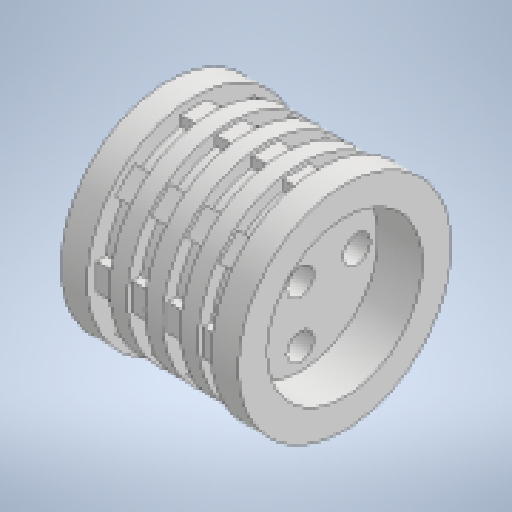
# Autodesk Inventor part: koła tak 1234
Saved by Autodesk Inventor 2023.5 (Build 275446000, 446)
## iProperties
Created: 2025-02-04
Part Number: koła tak 1234
Material: Ogólny
Document SubType Name: Modeling
Designer: idzim
Density: 1 g/cm^3
Appearance: Domyślna
Author: idzim
Autodesk Inventor part; units mm, degrees
ref_plane "YZ Plane" through (0, 0, 0) normal (1, 0, 0) x (0, 1, 0)
ref_plane "XZ Plane" through (0, 0, 0) normal (0, 1, 0) x (-1, 0, 0)
ref_plane "XY Plane" through (0, 0, 0) normal (0, 0, 1) x (1, 0, 0)
sketch "Szkic1" plane through (0, 0, 0) normal (1, 0, 0) x (0, 1, 0)
  circle A0 centre (0, 0) radius 15
  circle A1 centre (0, 0) radius 12
  circle A2 centre (0, 0) radius 10
  circle A3 centre (0, 0) radius 8.75
  dimension "d0" = 30
  dimension "d1" = 24
  dimension "d2" = 20
  dimension "d3" = 17.5
  constraints: 4 centre point, 4 coincident
  measures "d0" diameter of A0
  measures "d1" diameter of A1
  measures "d2" diameter of A2
  measures "d3" diameter of A3
extrude "Wyciągnięcie proste1" add sketch "Szkic1" along normal blind 3 contours A1 | A2 | A3
sketch "Szkic2" plane through (3, 0, 0) normal (1, 0, 0) x (0, 0, -1)
  circle A0 centre (0, 0) radius 8.75
  circle A1 centre (0, 0) radius 10
  circle A2 centre (0, 0) radius 11.25
  line L0 (1.5, 9) -> (-1.5, 9)
  line L1 (-1.5, 9) -> (-1.5, 11)
  line L2 (-1.5, 11) -> (1.5, 11)
  line L3 (1.5, 11) -> (1.5, 9)
  line L4 (1.5, 9) -> (-1.5, 11) construction
  line L5 (-1.5, 9) -> (1.5, 11) construction
  line L6 (-5.3033, 7.4246) -> (-7.4246, 5.3033)
  line L7 (-7.4246, 5.3033) -> (-8.8388, 6.7175)
  line L8 (-8.8388, 6.7175) -> (-6.7175, 8.8388)
  line L9 (-6.7175, 8.8388) -> (-5.3033, 7.4246)
  line L10 (-5.3033, 7.4246) -> (-8.8388, 6.7175) construction
  line L11 (-7.4246, 5.3033) -> (-6.7175, 8.8388) construction
  line L12 (-9, 1.5) -> (-9, -1.5)
  line L13 (-9, -1.5) -> (-11, -1.5)
  line L14 (-11, -1.5) -> (-11, 1.5)
  line L15 (-11, 1.5) -> (-9, 1.5)
  line L16 (-9, 1.5) -> (-11, -1.5) construction
  line L17 (-9, -1.5) -> (-11, 1.5) construction
  line L18 (-7.4246, -5.3033) -> (-5.3033, -7.4246)
  line L19 (-5.3033, -7.4246) -> (-6.7175, -8.8388)
  line L20 (-6.7175, -8.8388) -> (-8.8388, -6.7175)
  line L21 (-8.8388, -6.7175) -> (-7.4246, -5.3033)
  line L22 (-7.4246, -5.3033) -> (-6.7175, -8.8388) construction
  line L23 (-5.3033, -7.4246) -> (-8.8388, -6.7175) construction
  line L24 (-1.5, -9) -> (1.5, -9)
  line L25 (1.5, -9) -> (1.5, -11)
  line L26 (1.5, -11) -> (-1.5, -11)
  line L27 (-1.5, -11) -> (-1.5, -9)
  line L28 (-1.5, -9) -> (1.5, -11) construction
  line L29 (1.5, -9) -> (-1.5, -11) construction
  line L30 (5.3033, -7.4246) -> (7.4246, -5.3033)
  line L31 (7.4246, -5.3033) -> (8.8388, -6.7175)
  line L32 (8.8388, -6.7175) -> (6.7175, -8.8388)
  line L33 (6.7175, -8.8388) -> (5.3033, -7.4246)
  line L34 (5.3033, -7.4246) -> (8.8388, -6.7175) construction
  line L35 (7.4246, -5.3033) -> (6.7175, -8.8388) construction
  line L36 (9, -1.5) -> (9, 1.5)
  line L37 (9, 1.5) -> (11, 1.5)
  line L38 (11, 1.5) -> (11, -1.5)
  line L39 (11, -1.5) -> (9, -1.5)
  line L40 (9, -1.5) -> (11, 1.5) construction
  line L41 (9, 1.5) -> (11, -1.5) construction
  line L42 (7.4246, 5.3033) -> (5.3033, 7.4246)
  line L43 (5.3033, 7.4246) -> (6.7175, 8.8388)
  line L44 (6.7175, 8.8388) -> (8.8388, 6.7175)
  line L45 (8.8388, 6.7175) -> (7.4246, 5.3033)
  line L46 (7.4246, 5.3033) -> (6.7175, 8.8388) construction
  line L47 (5.3033, 7.4246) -> (8.8388, 6.7175) construction
  point P0 (0, 10)
  point P1 (-7.0711, 7.0711)
  point P2 (-10, 0)
  point P3 (-7.0711, -7.0711)
  point P4 (0, -10)
  point P5 (7.0711, -7.0711)
  point P6 (10, 0)
  point P7 (7.0711, 7.0711)
  point P8 (-1.5, 9.8869)
  point P9 (-5.9304, 8.0517)
  point P10 (-8.0517, 5.9304)
  point P11 (-9.8869, 1.5)
  point P12 (-9.8869, -1.5)
  point P13 (-8.0517, -5.9304)
  point P14 (-5.9304, -8.0517)
  point P15 (-1.5, -9.8869)
  point P16 (1.5, -9.8869)
  point P17 (5.9304, -8.0517)
  point P18 (8.0517, -5.9304)
  point P19 (9.8869, -1.5)
  point P20 (9.8869, 1.5)
  point P21 (8.0517, 5.9304)
  point P22 (5.9304, 8.0517)
  point P23 (1.5, 9.8869)
  dimension "d7" = 20
  dimension "d6" = 17.5
  dimension "d8" = 22.5
  dimension "d9" = 3
  dimension "d10" = 2
  dimension "d13" = 360
  constraints: 96 end point, 3 coincident, 2 centre point, 2 midpoint, 2 parallel, 1 horizontal, 1 perpendicular, 92 other
  measures "d6" diameter of A0
  measures "d8" diameter of A2
  measures "d9" distance of L1.end L2.end
  measures "d10" distance of L0.end L1.end
extrude "Wyciągnięcie proste2" add sketch "Szkic2" along normal blind 2 contours A0 | A1 L39 L36 L37 | A1 L37 L38 L39 | L37 L36 L39 A1 L31 L30 L33 L25 L24 L27 L19 L18 L21 L13 L12 L15 L7 L6 L9 L1 L0 L3 L43 L42 L45 | L45 L42 L43 A1 | A1 L43 L44 L45 | L31 L32 L33 A1 | A1 L33 L30 L31 | L3 L0 L1 A1 | A1 L1 L2 L3 | L25 L26 L27 A1 | A1 L27 L24 L25 | L9 L6 L7 A1 | A1 L7 L8 L9 | L19 L20 L21 A1 | A1 L21 L18 L19 | L15 L12 L13 A1 | A1 L13 L14 L15
sketch "Szkic3" plane through (5, 0, 0) normal (1, 0, 0) x (0, 0, -1)
  circle A0 centre (0, 0) radius 11.5
  dimension "d17" = 23
  constraints: 1 centre point, 1 coincident
  measures "d17" diameter of A0
extrude "Wyciągnięcie proste3" add sketch "Szkic3" along normal blind 2
sketch "Szkic4" plane through (7, 0, 0) normal (1, 0, 0) x (0, 0, -1)
  circle A0 centre (0, 0.0528) radius 8.75
  circle A1 centre (0, 0.0528) radius 10
  circle A2 centre (0, 0.0528) radius 11.25
  line L0 (1.5, 9.0528) -> (-1.5, 9.0528)
  line L1 (-1.5, 9.0528) -> (-1.5, 11.0528)
  line L2 (-1.5, 11.0528) -> (1.5, 11.0528)
  line L3 (1.5, 11.0528) -> (1.5, 9.0528)
  line L4 (1.5, 9.0528) -> (-1.5, 11.0528) construction
  line L5 (-1.5, 9.0528) -> (1.5, 11.0528) construction
  line L6 (-5.3033, 7.4774) -> (-7.4246, 5.3561)
  line L7 (-7.4246, 5.3561) -> (-8.8388, 6.7703)
  line L8 (-8.8388, 6.7703) -> (-6.7175, 8.8916)
  line L9 (-6.7175, 8.8916) -> (-5.3033, 7.4774)
  line L10 (-5.3033, 7.4774) -> (-8.8388, 6.7703) construction
  line L11 (-7.4246, 5.3561) -> (-6.7175, 8.8916) construction
  line L12 (-9, 1.5528) -> (-9, -1.4472)
  line L13 (-9, -1.4472) -> (-11, -1.4472)
  line L14 (-11, -1.4472) -> (-11, 1.5528)
  line L15 (-11, 1.5528) -> (-9, 1.5528)
  line L16 (-9, 1.5528) -> (-11, -1.4472) construction
  line L17 (-9, -1.4472) -> (-11, 1.5528) construction
  line L18 (-7.4246, -5.2505) -> (-5.3033, -7.3718)
  line L19 (-5.3033, -7.3718) -> (-6.7175, -8.7861)
  line L20 (-6.7175, -8.7861) -> (-8.8388, -6.6647)
  line L21 (-8.8388, -6.6647) -> (-7.4246, -5.2505)
  line L22 (-7.4246, -5.2505) -> (-6.7175, -8.7861) construction
  line L23 (-5.3033, -7.3718) -> (-8.8388, -6.6647) construction
  line L24 (-1.5, -8.9472) -> (1.5, -8.9472)
  line L25 (1.5, -8.9472) -> (1.5, -10.9472)
  line L26 (1.5, -10.9472) -> (-1.5, -10.9472)
  line L27 (-1.5, -10.9472) -> (-1.5, -8.9472)
  line L28 (-1.5, -8.9472) -> (1.5, -10.9472) construction
  line L29 (1.5, -8.9472) -> (-1.5, -10.9472) construction
  line L30 (5.3033, -7.3718) -> (7.4246, -5.2505)
  line L31 (7.4246, -5.2505) -> (8.8388, -6.6647)
  line L32 (8.8388, -6.6647) -> (6.7175, -8.7861)
  line L33 (6.7175, -8.7861) -> (5.3033, -7.3718)
  line L34 (5.3033, -7.3718) -> (8.8388, -6.6647) construction
  line L35 (7.4246, -5.2505) -> (6.7175, -8.7861) construction
  line L36 (9, -1.4472) -> (9, 1.5528)
  line L37 (9, 1.5528) -> (11, 1.5528)
  line L38 (11, 1.5528) -> (11, -1.4472)
  line L39 (11, -1.4472) -> (9, -1.4472)
  line L40 (9, -1.4472) -> (11, 1.5528) construction
  line L41 (9, 1.5528) -> (11, -1.4472) construction
  line L42 (7.4246, 5.3561) -> (5.3033, 7.4774)
  line L43 (5.3033, 7.4774) -> (6.7175, 8.8916)
  line L44 (6.7175, 8.8916) -> (8.8388, 6.7703)
  line L45 (8.8388, 6.7703) -> (7.4246, 5.3561)
  line L46 (7.4246, 5.3561) -> (6.7175, 8.8916) construction
  line L47 (5.3033, 7.4774) -> (8.8388, 6.7703) construction
  point P0 (0, 0)
  point P1 (0, 10.0528)
  point P2 (-7.0711, 7.1238)
  point P3 (-10, 0.0528)
  point P4 (-7.0711, -7.0183)
  point P5 (0, -9.9472)
  point P6 (7.0711, -7.0183)
  point P7 (10, 0.0528)
  point P8 (7.0711, 7.1238)
  point P9 (-9.8869, -1.4472)
  point P10 (-8.0517, -5.8776)
  point P11 (-5.9304, -7.9989)
  point P12 (-1.5, -9.8341)
  point P13 (1.5, -9.8341)
  point P14 (5.9304, -7.9989)
  point P15 (8.0517, -5.8776)
  point P16 (9.8869, -1.4472)
  point P17 (9.8869, 1.5528)
  point P18 (8.0517, 5.9832)
  point P19 (5.9304, 8.1045)
  point P20 (1.5, 9.9396)
  point P21 (-1.5, 9.9396)
  point P22 (-5.9304, 8.1045)
  point P23 (-8.0517, 5.9832)
  point P24 (-9.8869, 1.5528)
  dimension "d23" = 20
  dimension "d22" = 17.5
  dimension "d24" = 22.5
  dimension "d25" = 3
  dimension "d26" = 2
  dimension "d27" = 360
  constraints: 96 end point, 3 coincident, 2 centre point, 2 midpoint, 2 parallel, 1 horizontal, 1 perpendicular, 92 other
  measures "d22" diameter of A0
  measures "d24" diameter of A2
  measures "d25" distance of L1.end L2.end
  measures "d26" distance of L1.start L1.end
extrude "Wyciągnięcie proste4" add sketch "Szkic4" along normal blind 2 contours A0 | A1 L39 L36 L37 | A1 L37 L38 L39 | L37 L36 L39 A1 L31 L30 L33 L25 L24 L27 L19 L18 L21 L13 L12 L15 L7 L6 L9 L1 L0 L3 L43 L42 L45 | L45 L42 L43 A1 | A1 L43 L44 L45 | L31 L32 L33 A1 | A1 L33 L30 L31 | L3 L0 L1 A1 | A1 L1 L2 L3 | L25 L26 L27 A1 | A1 L27 L24 L25 | L9 L6 L7 A1 | A1 L7 L8 L9 | L19 L20 L21 A1 | A1 L21 L18 L19 | L15 L12 L13 A1 | A1 L13 L14 L15
sketch "Szkic5" plane through (9, 0, 0) normal (1, 0, 0) x (0, 0, -1)
  circle A0 centre (0, 0) radius 11.5
  dimension "d30" = 23
  constraints: 1 centre point, 1 coincident
  measures "d30" diameter of A0
extrude "Wyciągnięcie proste5" add sketch "Szkic5" along normal blind 2
sketch "Szkic6" plane through (11, 0, 0) normal (1, 0, 0) x (0, 0, -1)
  circle A0 centre (0, 0) radius 8.75
  circle A1 centre (0, 0) radius 10
  circle A2 centre (0, 0) radius 11.25
  line L0 (1.5203, 9) -> (-1.4797, 9)
  line L1 (-1.4797, 9) -> (-1.4797, 11)
  line L2 (-1.4797, 11) -> (1.5203, 11)
  line L3 (1.5203, 11) -> (1.5203, 9)
  line L4 (1.5203, 9) -> (-1.4797, 11) construction
  line L5 (-1.4797, 9) -> (1.5203, 11) construction
  line L6 (-5.2889, 7.4389) -> (-7.4103, 5.3176)
  line L7 (-7.4103, 5.3176) -> (-8.8245, 6.7318)
  line L8 (-8.8245, 6.7318) -> (-6.7032, 8.8532)
  line L9 (-6.7032, 8.8532) -> (-5.2889, 7.4389)
  line L10 (-5.2889, 7.4389) -> (-8.8245, 6.7318) construction
  line L11 (-7.4103, 5.3176) -> (-6.7032, 8.8532) construction
  line L12 (-9, 1.5203) -> (-9, -1.4797)
  line L13 (-9, -1.4797) -> (-11, -1.4797)
  line L14 (-11, -1.4797) -> (-11, 1.5203)
  line L15 (-11, 1.5203) -> (-9, 1.5203)
  line L16 (-9, 1.5203) -> (-11, -1.4797) construction
  line L17 (-9, -1.4797) -> (-11, 1.5203) construction
  line L18 (-7.4389, -5.2889) -> (-5.3176, -7.4103)
  line L19 (-5.3176, -7.4103) -> (-6.7318, -8.8245)
  line L20 (-6.7318, -8.8245) -> (-8.8532, -6.7032)
  line L21 (-8.8532, -6.7032) -> (-7.4389, -5.2889)
  line L22 (-7.4389, -5.2889) -> (-6.7318, -8.8245) construction
  line L23 (-5.3176, -7.4103) -> (-8.8532, -6.7032) construction
  line L24 (-1.5203, -9) -> (1.4797, -9)
  line L25 (1.4797, -9) -> (1.4797, -11)
  line L26 (1.4797, -11) -> (-1.5203, -11)
  line L27 (-1.5203, -11) -> (-1.5203, -9)
  line L28 (-1.5203, -9) -> (1.4797, -11) construction
  line L29 (1.4797, -9) -> (-1.5203, -11) construction
  line L30 (5.2889, -7.4389) -> (7.4103, -5.3176)
  line L31 (7.4103, -5.3176) -> (8.8245, -6.7318)
  line L32 (8.8245, -6.7318) -> (6.7032, -8.8532)
  line L33 (6.7032, -8.8532) -> (5.2889, -7.4389)
  line L34 (5.2889, -7.4389) -> (8.8245, -6.7318) construction
  line L35 (7.4103, -5.3176) -> (6.7032, -8.8532) construction
  line L36 (9, -1.5203) -> (9, 1.4797)
  line L37 (9, 1.4797) -> (11, 1.4797)
  line L38 (11, 1.4797) -> (11, -1.5203)
  line L39 (11, -1.5203) -> (9, -1.5203)
  line L40 (9, -1.5203) -> (11, 1.4797) construction
  line L41 (9, 1.4797) -> (11, -1.5203) construction
  line L42 (7.4389, 5.2889) -> (5.3176, 7.4103)
  line L43 (5.3176, 7.4103) -> (6.7318, 8.8245)
  line L44 (6.7318, 8.8245) -> (8.8532, 6.7032)
  line L45 (8.8532, 6.7032) -> (7.4389, 5.2889)
  line L46 (7.4389, 5.2889) -> (6.7318, 8.8245) construction
  line L47 (5.3176, 7.4103) -> (8.8532, 6.7032) construction
  point P0 (0, 0)
  point P1 (0.0203, 10)
  point P2 (-7.0567, 7.0854)
  point P3 (-10, 0.0203)
  point P4 (-7.0854, -7.0567)
  point P5 (-0.0203, -10)
  point P6 (7.0567, -7.0854)
  point P7 (10, -0.0203)
  point P8 (7.0854, 7.0567)
  point P9 (-1.4797, 9.8899)
  point P10 (-5.9139, 8.0639)
  point P11 (-8.0395, 5.9469)
  point P12 (-9.8838, 1.5203)
  point P13 (-9.8899, -1.4797)
  point P14 (-8.0639, -5.9139)
  point P15 (-5.9469, -8.0395)
  point P16 (-1.5203, -9.8838)
  point P17 (1.4797, -9.8899)
  point P18 (5.9139, -8.0639)
  point P19 (8.0395, -5.9469)
  point P20 (9.8838, -1.5203)
  point P21 (9.8899, 1.4797)
  point P22 (8.0639, 5.9139)
  point P23 (5.9469, 8.0395)
  point P24 (1.5203, 9.8838)
  dimension "d13" = 360
  dimension "d36" = 20
  dimension "d35" = 17.5
  dimension "d37" = 22.5
  dimension "d38" = 3
  dimension "d39" = 2
  dimension "d40" = 360
  constraints: 96 end point, 4 coincident, 2 centre point, 2 midpoint, 2 parallel, 1 horizontal, 1 perpendicular, 92 other
  measures "d35" diameter of A0
  measures "d37" diameter of A2
  measures "d38" distance of L1.end L2.end
  measures "d39" distance of L1.start L1.end
extrude "Wyciągnięcie proste6" add sketch "Szkic6" along normal blind 2 contours A0 | A1 L39 L36 L37 | A1 L37 L38 L39 | L37 L36 L39 A1 L31 L30 L33 L25 L24 L27 L19 L18 L21 L13 L12 L15 L7 L6 L9 L1 L0 L3 L43 L42 L45 | L45 L42 L43 A1 | A1 L43 L44 L45 | L31 L32 L33 A1 | A1 L33 L30 L31 | L3 L0 L1 A1 | A1 L1 L2 L3 | L25 L26 L27 A1 | A1 L27 L24 L25 | L9 L6 L7 A1 | A1 L7 L8 L9 | L19 L20 L21 A1 | A1 L21 L18 L19 | L15 L12 L13 A1 | A1 L13 L14 L15
sketch "Szkic7" plane through (13, 0, 0) normal (1, 0, 0) x (0, 0, -1)
  circle A0 centre (0, 0) radius 11.5
  dimension "d44" = 23
  constraints: 1 centre point, 1 coincident
  measures "d44" diameter of A0
extrude "Wyciągnięcie proste7" add sketch "Szkic7" along normal blind 2
sketch "Szkic8" plane through (15, 0, 0) normal (1, 0, 0) x (0, 0, -1)
  circle A0 centre (0, 0) radius 8.75
  circle A1 centre (0, 0) radius 10
  circle A2 centre (0, 0) radius 11.25
  line L0 (1.0323, 8.9891) -> (-1.9677, 8.9891)
  line L1 (-1.9677, 8.9891) -> (-1.9677, 10.9891)
  line L2 (-1.9677, 10.9891) -> (1.0323, 10.9891)
  line L3 (1.0323, 10.9891) -> (1.0323, 8.9891)
  line L4 (1.0323, 8.9891) -> (-1.9677, 10.9891) construction
  line L5 (-1.9677, 8.9891) -> (1.0323, 10.9891) construction
  line L6 (-5.6263, 7.0862) -> (-7.7476, 4.9648)
  line L7 (-7.7476, 4.9648) -> (-9.1618, 6.3791)
  line L8 (-9.1618, 6.3791) -> (-7.0405, 8.5004)
  line L9 (-7.0405, 8.5004) -> (-5.6263, 7.0862)
  line L10 (-5.6263, 7.0862) -> (-9.1618, 6.3791) construction
  line L11 (-7.7476, 4.9648) -> (-7.0405, 8.5004) construction
  line L12 (-8.9891, 1.0323) -> (-8.9891, -1.9677)
  line L13 (-8.9891, -1.9677) -> (-10.9891, -1.9677)
  line L14 (-10.9891, -1.9677) -> (-10.9891, 1.0323)
  line L15 (-10.9891, 1.0323) -> (-8.9891, 1.0323)
  line L16 (-8.9891, 1.0323) -> (-10.9891, -1.9677) construction
  line L17 (-8.9891, -1.9677) -> (-10.9891, 1.0323) construction
  line L18 (-7.0862, -5.6263) -> (-4.9648, -7.7476)
  line L19 (-4.9648, -7.7476) -> (-6.3791, -9.1618)
  line L20 (-6.3791, -9.1618) -> (-8.5004, -7.0405)
  line L21 (-8.5004, -7.0405) -> (-7.0862, -5.6263)
  line L22 (-7.0862, -5.6263) -> (-6.3791, -9.1618) construction
  line L23 (-4.9648, -7.7476) -> (-8.5004, -7.0405) construction
  line L24 (-1.0323, -8.9891) -> (1.9677, -8.9891)
  line L25 (1.9677, -8.9891) -> (1.9677, -10.9891)
  line L26 (1.9677, -10.9891) -> (-1.0323, -10.9891)
  line L27 (-1.0323, -10.9891) -> (-1.0323, -8.9891)
  line L28 (-1.0323, -8.9891) -> (1.9677, -10.9891) construction
  line L29 (1.9677, -8.9891) -> (-1.0323, -10.9891) construction
  line L30 (5.6263, -7.0862) -> (7.7476, -4.9648)
  line L31 (7.7476, -4.9648) -> (9.1618, -6.3791)
  line L32 (9.1618, -6.3791) -> (7.0405, -8.5004)
  line L33 (7.0405, -8.5004) -> (5.6263, -7.0862)
  line L34 (5.6263, -7.0862) -> (9.1618, -6.3791) construction
  line L35 (7.7476, -4.9648) -> (7.0405, -8.5004) construction
  line L36 (8.9891, -1.0323) -> (8.9891, 1.9677)
  line L37 (8.9891, 1.9677) -> (10.9891, 1.9677)
  line L38 (10.9891, 1.9677) -> (10.9891, -1.0323)
  line L39 (10.9891, -1.0323) -> (8.9891, -1.0323)
  line L40 (8.9891, -1.0323) -> (10.9891, 1.9677) construction
  line L41 (8.9891, 1.9677) -> (10.9891, -1.0323) construction
  line L42 (7.0862, 5.6263) -> (4.9648, 7.7476)
  line L43 (4.9648, 7.7476) -> (6.3791, 9.1618)
  line L44 (6.3791, 9.1618) -> (8.5004, 7.0405)
  line L45 (8.5004, 7.0405) -> (7.0862, 5.6263)
  line L46 (7.0862, 5.6263) -> (6.3791, 9.1618) construction
  line L47 (4.9648, 7.7476) -> (8.5004, 7.0405) construction
  point P0 (0, 0)
  point P1 (-0.4677, 9.9891)
  point P2 (-7.3941, 6.7326)
  point P3 (-9.9891, -0.4677)
  point P4 (-6.7326, -7.3941)
  point P5 (0.4677, -9.9891)
  point P6 (7.3941, -6.7326)
  point P7 (9.9891, 0.4677)
  point P8 (6.7326, 7.3941)
  point P9 (-1.9677, 9.8045)
  point P10 (-6.3034, 7.7632)
  point P11 (-8.3242, 5.5414)
  point P12 (-9.9466, 1.0323)
  point P13 (-9.8045, -1.9677)
  point P14 (-7.7632, -6.3034)
  point P15 (-5.5414, -8.3242)
  point P16 (-1.0323, -9.9466)
  point P17 (1.9677, -9.8045)
  point P18 (6.3034, -7.7632)
  point P19 (8.3242, -5.5414)
  point P20 (9.9466, -1.0323)
  point P21 (9.8045, 1.9677)
  point P22 (7.7632, 6.3034)
  point P23 (5.5414, 8.3242)
  point P24 (1.0323, 9.9466)
  dimension "d50" = 20
  dimension "d49" = 17.5
  dimension "d51" = 22.5
  dimension "d52" = 3
  dimension "d53" = 2
  dimension "d54" = 360
  constraints: 96 end point, 4 coincident, 2 centre point, 2 midpoint, 2 parallel, 1 horizontal, 1 perpendicular, 92 other
  measures "d49" diameter of A0
  measures "d51" diameter of A2
  measures "d52" distance of L1.end L2.end
  measures "d53" distance of L1.start L1.end
extrude "Wyciągnięcie proste8" add sketch "Szkic8" along normal blind 2 contours A0 | A1 L39 L36 L37 | A1 L37 L38 L39 | L37 L36 L39 A1 L31 L30 L33 L25 L24 L27 L19 L18 L21 L13 L12 L15 L7 L6 L9 L1 L0 L3 L43 L42 L45 | L45 L42 L43 A1 | A1 L43 L44 L45 | L31 L32 L33 A1 | A1 L33 L30 L31 | L3 L0 L1 A1 | A1 L1 L2 L3 | L25 L26 L27 A1 | A1 L27 L24 L25 | L9 L6 L7 A1 | A1 L7 L8 L9 | L19 L20 L21 A1 | A1 L21 L18 L19 | L15 L12 L13 A1 | A1 L13 L14 L15
sketch "Szkic9" plane through (17, 0, 0) normal (1, 0, 0) x (0, 0, -1)
  circle A0 centre (0, 0) radius 12
  dimension "d57" = 24
  constraints: 1 centre point, 1 coincident
  measures "d57" diameter of A0
extrude "Wyciągnięcie proste9" add sketch "Szkic9" along normal blind 3
sketch "Szkic10" plane through (20, 0, 0) normal (1, 0, 0) x (0, 0, -1)
  circle A0 centre (0, 0) radius 8.75
  dimension "d60" = 17.5
  constraints: 1 centre point, 1 coincident
  measures "d60" diameter of A0
extrude "Wyciągnięcie proste10" cut sketch "Szkic10" against normal blind 5
sketch "Szkic11" plane through (15, 0, 0) normal (1, 0, 0) x (0, 0, -1)
  circle A0 centre (0, 6.357) radius 1.5
  circle A1 centre (-6.357, 0) radius 1.5
  circle A2 centre (0, -6.357) radius 1.5
  circle A3 centre (6.357, 0) radius 1.5
  point P0 (0, 0)
  dimension "d63" = 3
  dimension "d64" = 6.357
  dimension "d67" = 360
  constraints: 4 centre point, 9 other
  measures "d63" diameter of A0
  measures "d64" distance of point (0, 0) A0.centre
extrude "Wyciągnięcie proste11" cut sketch "Szkic11" against normal blind 20
sketch "Szkic12" plane through (15, 0, 0) normal (1, 0, 0) x (0, 0, -1)
  circle A0 centre (0, 0) radius 1.5
  dimension "d71" = 3
  constraints: 1 centre point, 1 coincident
  measures "d71" diameter of A0
extrude "Wyciągnięcie proste12" cut sketch "Szkic12" against normal blind 5
sketch "Szkic25" plane through (0, 0, 0) normal (-1, 0, 0) x (0, 0, 1)
  circle A0 centre (0, 0) radius 9.557
  circle A1 centre (-6.357, 0) radius 1.5 projected
  circle A2 centre (-6.357, 0) radius 3.2
  circle A3 centre (0, -6.357) radius 3.2
  circle A4 centre (6.357, 0) radius 3.2
  circle A5 centre (0, 6.357) radius 3.2
  dimension "d130" = 6.4
  dimension "d133" = 360
  constraints: 5 centre point, 4 coincident, 1 tangent, 11 other
  measures "d130" diameter of A2
extrude "Wyciągnięcie proste23" cut sketch "Szkic25" against normal blind 4 contours A5 | A2 | A3 | A4
chamfer "Faza2" distance 1 angle 45 4 edges at (0, 0, -9.557) (0, 6.357, -3.2) (0, 0, 3.157) (0, -6.357, -3.2)
